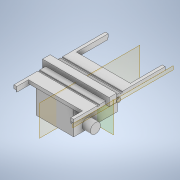
# Autodesk Inventor part: SAW_DM
Saved by Autodesk Inventor 2020 (Build 240168000, 168)
## iProperties
Created: 2020-01-03
Part Number: SAW_DM
Material: Générique
Document SubType Name: Modeling
Designer: damien
Density: 1 g/cm^3
Appearance: Par défaut
Author: damien
Autodesk Inventor part; units mm, degrees
ref_plane "YZ Plane" through (0, 0, 0) normal (1, 0, 0) x (0, 1, 0)
ref_plane "XZ Plane" through (0, 0, 0) normal (0, 1, 0) x (-1, 0, 0)
ref_plane "XY Plane" through (0, 0, 0) normal (0, 0, 1) x (1, 0, 0)
sketch "Esquisse1" plane through (0, 0, 0) normal (0, 1, 0) x (-1, 0, 0)
  line L0 (-225, -262.5) -> (225, -262.5)
  line L1 (225, -262.5) -> (225, 262.5)
  line L2 (225, 262.5) -> (-225, 262.5)
  line L3 (-225, 262.5) -> (-225, -262.5)
  line L4 (-225, -262.5) -> (225, 262.5) construction
  line L5 (225, -262.5) -> (-225, 262.5) construction
  point P0 (0, 0)
  dimension "d0" = 525
  dimension "d1" = 450
  constraints: 12 end point, 2 midpoint, 2 parallel, 1 horizontal, 1 perpendicular
  measures "d0" distance of L0.end L1.end
  measures "d1" distance of L1.end L2.end
extrude "Extrusion1" add sketch "Esquisse1" along normal blind 290
sketch "Esquisse2" plane through (0, 290, 0) normal (0, 1, 0) x (1, 0, 0)
  line L0 (-343, 683) -> (-343, -410)
  line L1 (-343, -410) -> (-308, -410)
  line L2 (373, -410) -> (373, 683)
  line L3 (-308, -410) -> (-308, -271)
  line L4 (-308, -271) -> (338, -271)
  line L5 (338, -271) -> (338, -410)
  line L6 (-308, 683) -> (-308, 302)
  line L7 (-308, 302) -> (338, 302)
  line L8 (338, 302) -> (338, 683)
  line L9 (373, 683) -> (338, 683)
  line L10 (-308, 683) -> (-343, 683)
  line L11 (338, -410) -> (373, -410)
  line L12 (-225, 262.5) -> (-225, -262.5) construction
  line L13 (225, -262.5) -> (225, 262.5) construction
  line L14 (225, 262.5) -> (-225, 262.5) construction
  line L15 (-225, -262.5) -> (225, -262.5) construction
  point P0 (0, 0)
  dimension "d4" = 646
  dimension "d5" = 573
  dimension "d6" = 139
  dimension "d7" = 381
  dimension "d8" = 35
  dimension "d9" = 35
  dimension "d10" = 118
  dimension "d11" = 148
  dimension "d12" = 1093
  dimension "d13" = 39.5
  dimension "d14" = 8.5
  dimension "d15" = 525
  constraints: 24 end point, 7 perpendicular, 4 collinear, 3 horizontal, 3 parallel, 2 vertical
  measures "d4" distance of L3.end L4.end
  measures "d5" distance between parallel lines of L7 L4
  measures "d6" distance of L1.end L3.end
  measures "d7" distance of L6.start L6.end
  measures "d8" distance between parallel lines of L5 L2
  measures "d9" distance of L6.start L0.start
  measures "d10" distance between parallel lines of L12 L0
  measures "d11" distance between parallel lines of L2 L13
  measures "d12" distance of L0.start L0.end
  measures "d13" distance between parallel lines of L14 L7
  measures "d14" distance between parallel lines of L15 L4
  measures "d15" distance of L13.start L13.end
extrude "Extrusion2" add sketch "Esquisse2" along normal blind 40
sketch "Esquisse3" plane through (338, 290, 410) normal (0, 0, 1) x (1, 0, 0)
  line L0 (-646, 0) -> (0, 0) projected
  line L1 (-646, 0) -> (-649, 0)
  line L2 (-649, 0) -> (-649, -19)
  line L3 (-649, -19) -> (-646, -19)
  line L4 (-646, -19) -> (-646, 0)
  line L5 (0, 0) -> (35, 0) projected
  line L6 (0, 0) -> (3, 0)
  line L7 (3, 0) -> (3, -19)
  line L8 (3, -19) -> (0, -19)
  line L9 (0, -19) -> (0, 0)
  line L10 (0, 40) -> (35, 40) projected
  point P0 (-338, -290)
  point P1 (3, 0)
  dimension "d18" = 59
  dimension "d19" = 3
  constraints: 16 end point, 4 parallel, 2 collinear, 2 horizontal, 2 perpendicular
  measures "d18" distance between parallel lines of L10 L8
  measures "d19" distance of L7.end L8.end
extrude "Extrusion3" add sketch "Esquisse3" against normal blind 1090
sketch "Esquisse4" plane through (-225, 0, -262.5) normal (-1, 0, 0) x (0, 0, 1)
  circle A0 centre (255, 80) radius 40
  line L0 (0, 0) -> (0, 290) projected
  line L1 (0, 0) -> (525, 0) projected
  line L2 (525, 0) -> (525, 290) projected
  point P0 (262.5, 0)
  dimension "d23" = 80
  dimension "d24" = 255
  dimension "d25" = 80
  dimension "d26" = 270
  constraints: 1 centre point
  measures "d23" diameter of A0
  measures "d24" distance from line of L0 A0.centre
  measures "d25" distance from line of A0.centre L1
  measures "d26" distance from line of L2 A0.centre
extrude "Extrusion4" add sketch "Esquisse4" along normal blind 110
sketch "Esquisse5" plane through (225, 0, -262.5) normal (0, 0, -1) x (-1, 0, 0)
  line L0 (0, 0) -> (0, 290) projected
  line L1 (0, 290) -> (110, 290)
  line L2 (110, 290) -> (110, 200)
  line L3 (110, 200) -> (0, 200)
  line L4 (0, 200) -> (0, 290)
  point P0 (225, 0)
  point P1 (0, 200)
  dimension "d29" = 90
  dimension "d30" = 110
  constraints: 8 end point, 2 parallel, 1 horizontal, 1 perpendicular
  measures "d29" distance of L1.end L2.end
  measures "d30" distance of L2.end L3.end
extrude "Extrusion5" add sketch "Esquisse5" along normal blind 30
sketch "Esquisse6" plane through (225, 0, 262.5) normal (1, 0, 0) x (0, 0, -1)
  circle A0 centre (160, 60) radius 60
  line L0 (0, 0) -> (0, 290) projected
  line L1 (0, 0) -> (525, 0) projected
  point P0 (262.5, 0)
  dimension "d33" = 120
  dimension "d34" = 160
  dimension "d35" = 60
  constraints: 1 centre point
  measures "d33" diameter of A0
  measures "d34" distance from line of L0 A0.centre
  measures "d35" distance from line of L1 A0.centre
extrude "Extrusion6" add sketch "Esquisse6" along normal blind 100
sketch "Esquisse8" plane through (225, 0, 262.5) normal (1, 0, 0) x (0, 0, -1)
  circle A0 centre (380, 271) radius 25
  line L0 (525, 0) -> (525, 200) projected
  line L1 (-147.5, 271) -> (942.5, 271) projected
  point P0 (262.5, 0)
  dimension "d38" = 50
  dimension "d39" = 145
  constraints: 1 centre point, 1 point on line
  measures "d38" diameter of A0
  measures "d39" distance from line of L0 A0.centre
extrude "Extrusion7" add sketch "Esquisse8" along normal blind 160
sketch "Esquisse9" plane through (-225, 0, -262.5) normal (-1, 0, 0) x (0, 0, 1)
  arc A0 (128.7519, 290) -> (161.2481, 290) centre (145, 271) ccw projected
  circle A1 centre (145, 271) radius 22.5
  point P0 (262.5, 0)
  dimension "d42" = 45
  constraints: 1 centre point, 1 coincident
  measures "d42" diameter of A1
extrude "Extrusion8" add sketch "Esquisse9" along normal blind 110
ref_plane "Plan de construction1" through (15, 290, -683) normal (1, 0, 0) x (0, 0, -1)
ref_plane "Plan de construction2" through (338, 290, -15.5) normal (0, 0, -1) x (-1, 0, 0)
ref_plane "Plan de construction3" through (413, 290, -683) normal (1, 0, 0) x (0, 0, -1)
sketch "Esquisse10" plane through (413, 290, -683) normal (1, 0, 0) x (0, 0, -1)
  line L0 (-620.5, 0) -> (-710.5, 0)
  line L1 (-710.5, 0) -> (-710.5, 95)
  line L2 (-710.5, 95) -> (-620.5, 95)
  line L3 (-620.5, 95) -> (-620.5, 0)
  line L4 (-549.2519, 0) -> (0, 0) projected
  line L5 (-390.5, 0) -> (-390.5, -90) projected
  line L6 (-420.5, -290) -> (-420.5, -90) projected
  point P0 (-683, -290)
  dimension "d46" = 90
  dimension "d47" = 95
  dimension "d50" = 200
  constraints: 8 end point, 2 parallel, 1 collinear, 1 horizontal, 1 perpendicular
  measures "d46" distance of L0.start L0.end
  measures "d47" distance of L2.end L0.start
  measures "d50" distance between parallel lines of L3 L6
extrude "Extrusion9" add sketch "Esquisse10" against normal blind 796
sketch "Esquisse11" plane through (-343, 290, -683) normal (-1, 0, 0) x (0, 0, 1)
  line L0 (577.552, 0) -> (945.5, 0) projected
  line L1 (785, 40) -> (809, 40)
  line L2 (809, 40) -> (809, 29)
  line L3 (809, 29) -> (785, 29)
  line L4 (785, 29) -> (785, 40)
  line L5 (945.5, -290) -> (945.5, 0) projected
  line L6 (710.5, 40) -> (1093, 40) projected
  line L7 (620.5, 40) -> (0, 40) projected
  line L8 (512, 40) -> (536, 40)
  line L9 (536, 40) -> (536, 29)
  line L10 (536, 29) -> (512, 29)
  line L11 (512, 29) -> (512, 40)
  line L12 (420.5, -290) -> (420.5, 0) projected
  line L13 (381, 0) -> (381, 40) projected
  point P0 (683, -290)
  point P1 (954, 40)
  dimension "d52" = 24
  dimension "d53" = 11
  dimension "d57" = 131
  dimension "d58" = 145
  constraints: 16 end point, 4 parallel, 3 collinear, 2 horizontal, 2 perpendicular, 1 point on line
  measures "d52" distance of L2.end L3.end
  measures "d53" distance of L1.end L2.end
  measures "d57" distance between parallel lines of L13 L11
  measures "d58" distance from line of point (954, 40) L2
extrude "Extrusion10" cut sketch "Esquisse11" against normal blind 776
